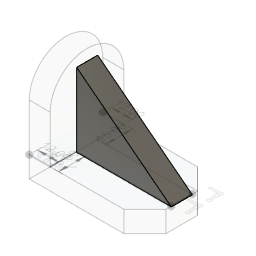
A1 (Autodesk Fusion 360 design; units mm, degrees)
Autodesk Fusion 360 part; units mm, degrees
note: some values were not read from the file. Chosen so that the rebuilt part matches the saved one: which pieces of a blend or face edit are solid.
sketch "Sketch1" plane through (0, 0, 0) normal (0, 0, 1) x (1, 0, 0)
  line L0 (50, 50) -> (104, 50)
  line L1 (116, 62) -> (104, 50)
  line L2 (116, 62) -> (116, 80)
  line L3 (50, 50) -> (50, 92)
  line L4 (50, 92) -> (104, 92)
  line L5 (104, 92) -> (116, 80)
  constraint horizontal L0
  constraint perpendicular L0 L3
  constraint perpendicular L3 L4
  constraint perpendicular L1 L5
extrude "Extrude1" add sketch "Sketch1" along normal blind 12 makes body 1
sketch "Sketch2" plane through (0, 0, 12) normal (0, 0, 1) x (-1, 0, 0)
  line L0 (-50, -50) -> (-104, -50)
  line L1 (-104, -50) -> (-116, -62)
  line L2 (-116, -62) -> (-116, -80)
  line L3 (-116, -80) -> (-104, -92)
  line L4 (-104, -92) -> (-50, -92)
  line L5 (-50, -92) -> (-50, -50)
  line L6 (-50, -50) -> (-62, -50)
  line L7 (-62, -50) -> (-62, -65)
  line L8 (-62, -65) -> (-116, -65)
  line L9 (-50, -92) -> (-62, -92)
  line L10 (-62, -92) -> (-62, -77)
  line L11 (-62, -77) -> (-116, -77)
  line L12 (-116, -77) -> (-116, -65)
  line L13 (-62, -77) -> (-62, -65)
  dimension "d22" = 12
  dimension "d23" = 15
  dimension "d24" = 12
  dimension "d27" = 15
  constraint coincident L0.start L5.end
  constraint perpendicular L5 L6
  constraint perpendicular L0 L7
  constraint coincident L2 L8.end
  constraint perpendicular L2 L8
  constraint coincident L4.end L5.start
  constraint perpendicular L5 L9
  constraint perpendicular L9 L10
  constraint coincident L2 L11.end
  constraint perpendicular L2 L11
  measures "d22" distance of L0.start L6.end
  measures "d23" distance of L6.end L7.end
  measures "d24" distance of L4.end L9.end
  measures "d27" distance of L9.end L10.end
extrude "Extrude4" add sketch "Sketch2" along normal blind 48 contours L0 L4 L5 L6 L7 L9 L10 L13 bodies 1
extrude "Extrude3" add sketch "Sketch2" along normal blind 12 contours L0 L4 L5 L6 L7 L9 L10 L13 bodies 1
extrude "Extrude2" add sketch "Sketch2" along normal blind 12 contours L0 L4 L5 L6 L7 L9 L10 L13 bodies 1
fillet "Fillet1" radius 21 2 edges at (56, 50, 60) (56, 92, 60) 1 faces at (58, 78, 60) on bodies 1
sketch "Sketch1 (2)" plane through (0, 0, 0) normal (0, 1, 0) x (1, 0, 0) in component "Component"
  line L0 (62, -12) -> (62, -54)
  line L1 (62, -54) -> (116, -12)
  line L2 (116, -12) -> (62, -12)
  dimension "d37" = 42
  constraint vertical L0
  constraint perpendicular L0 L2
  measures "d37" distance of L0.start L0.end
extrude "Extrude1'" add sketch "Sketch1 (2)" along normal mid plane 12 separate body makes body 2 in component "Component"
component "Component" placed x (1, 0, 0) y (0, 1, 0) z (0, 0, 1) at (0, 0, 0)
equation "d32 = 60 mm - 12 mm"
